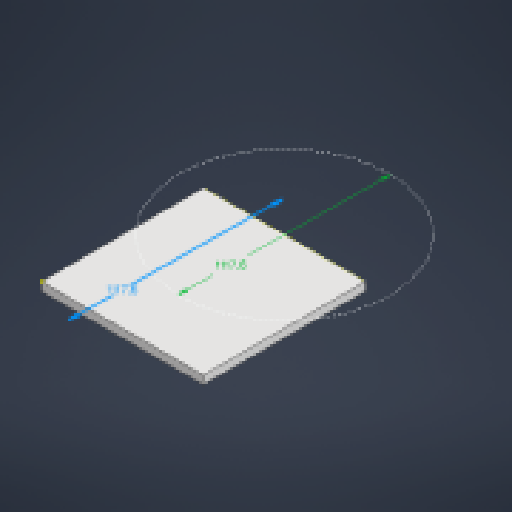
# Autodesk Inventor part: TableTop
Saved by Autodesk Inventor 2025 (Build 290162010, 162A)
## iProperties
Created: 2025-12-03
Part Number: TableTop
Material: Generic
Document SubType Name: Modeling
Designer: FizzyApple12
Density: 1 g/cm^3
Appearance: Default
Author: FizzyApple12
Autodesk Inventor part; units mm, degrees
ref_plane "YZ Plane" through (0, 0, 0) normal (1, 0, 0) x (0, 1, 0)
ref_plane "XZ Plane" through (0, 0, 0) normal (0, 1, 0) x (-1, 0, 0)
ref_plane "XY Plane" through (0, 0, 0) normal (0, 0, 1) x (1, 0, 0)
sketch "Sketch1" plane through (0, 0, 0) normal (0, 1, 0) x (-1, 0, 0)
  line L0 (0, 0) -> (-860.425, 0)
  line L1 (-860.425, 0) -> (-860.425, -860.425)
  line L2 (-860.425, -860.425) -> (0, -860.425)
  line L3 (0, -860.425) -> (0, 0)
  dimension "d0" = 860.425
  dimension "d1" = 860.425
  constraints: 8 end point, 2 parallel, 1 horizontal, 1 perpendicular
  measures "d0" distance of L2.end L1.end
  measures "d1" distance of L1.end L0.end
extrude "Extrusion1" add sketch "Sketch1" against normal blind 44.45
sketch "Sketch2" plane through (0, 0, 0) normal (0, 1, 0) x (1, 0, 0)
  line L0 (0, 860.425) -> (860.425, 860.425) construction
  circle A0 centre (430.2125, 860.425) radius 558.8 construction
  point P0 (0, 0)
  dimension "d4" = 1117.6
  constraints: 1 centre point, 1 midpoint
  measures "d4" diameter of A0
body "Solid1"
